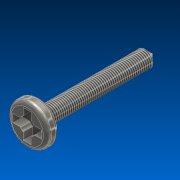
# Autodesk Inventor part: parafuso interno da ponte
Saved by Autodesk Inventor 2016 (Build 200138000, 138)
## iProperties
Created: 2018-12-10
Part Number: parafuso interno da ponte
Material: Generic
Document SubType Name: Modeling
Designer: lesly
Density: 1 g/cm^3
Appearance: Steel - Polished
Author: lesly
Autodesk Inventor part; units mm, degrees
ref_plane "YZ Plane" through (0, 0, 0) normal (1, 0, 0) x (0, 1, 0)
ref_plane "XZ Plane" through (0, 0, 0) normal (0, 1, 0) x (-1, 0, 0)
ref_plane "XY Plane" through (0, 0, 0) normal (0, 0, 1) x (1, 0, 0)
sketch "Sketch1" plane through (0, 0, 0) normal (0, 1, 0) x (-1, 0, 0)
  circle A0 centre (0, 0) radius 1
  dimension "d0" = 2
  constraints: 1 centre point
  measures "d0" diameter of A0
extrude "Extrusion1" add sketch "Sketch1" along normal blind 14
sketch "Sketch2" plane through (0, 0, 0) normal (0, -1, 0) x (1, 0, 0)
  circle A0 centre (0, 0) radius 2.5
  constraints: 1 centre point, 1 coincident
extrude "Extrusion2" add sketch "Sketch2" along normal blind 1.5
fillet "Fillet1" radius 0.5 2 edges at (-2.5, -1.5, 0) (-2.5, 0, 0)
sketch "Sketch3" plane through (0, -1.5, 0) normal (0, -1, 0) x (1, 0, 0)
  line L0 (1.75, -0.5) -> (1.75, 0.5)
  line L1 (-1.75, 0.5) -> (-1.75, -0.5)
  line L2 (0.5, 1.75) -> (-0.5, 1.75)
  line L3 (-0.5, -1.75) -> (0.5, -1.75)
  line L4 (1.75, 0.5) -> (0.866, 0.5)
  line L5 (-0.866, 0.5) -> (-1.75, 0.5)
  line L6 (-0.5, 1.75) -> (-0.5, 0.866)
  line L7 (-0.5, -0.866) -> (-0.5, -1.75)
  line L8 (0.5, 0.866) -> (0.5, 1.75)
  line L9 (-1.75, -0.5) -> (-0.866, -0.5)
  line L10 (0.866, -0.5) -> (1.75, -0.5)
  line L11 (0.5, -1.75) -> (0.5, -0.866)
  arc A0 (-0.5, 0.866) -> (-0.866, 0.5) centre (0, 0) ccw
  arc A1 (0.866, 0.5) -> (0.5, 0.866) centre (0, 0) ccw
  arc A2 (-0.866, -0.5) -> (-0.5, -0.866) centre (0, 0) ccw
  arc A3 (0.5, -0.866) -> (0.866, -0.5) centre (0, 0) ccw
  constraints: 24 end point, 10 parallel, 8 point on circle, 4 centre point, 4 perpendicular, 2 horizontal
extrude "Extrusion3" cut sketch "Sketch3" against normal blind 1.2
chamfer "Chamfer1" distance 1 angle 45 1 edges at (1, 14, 0)
thread "Thread1" size "M2x0.25" class "6g" standard "ANSI Metric M Profile" full length
body "Solid1"
